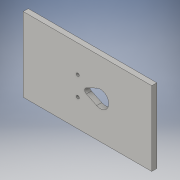
# Autodesk Inventor part: MOTORTOP
Saved by Autodesk Inventor 2016 (Build 200138000, 138)
## iProperties
Created: 2019-01-23
Part Number: MOTORTOP
Material: Generic
Document SubType Name: Modeling
Designer: student
Density: 1 g/cm^3
Appearance: Default
Author: student
Autodesk Inventor part; units mm, degrees
ref_plane "YZ Plane" through (0, 0, 0) normal (1, 0, 0) x (0, 1, 0)
ref_plane "XZ Plane" through (0, 0, 0) normal (0, 1, 0) x (-1, 0, 0)
ref_plane "XY Plane" through (0, 0, 0) normal (0, 0, 1) x (1, 0, 0)
sketch "Sketch1" plane through (0, 0, 0) normal (0, 0, 1) x (1, 0, 0)
  circle A0 centre (0, 0) radius 6.35 construction
  line L0 (0, 6.35) -> (-19.05, 6.35) construction
  circle A1 centre (-11.684, 0) radius 1.905 construction
  line L1 (-11.684, 0) -> (-19.05, 0) construction
  line L2 (-19.05, 0) -> (-20.3962, 0) construction
  line L3 (-20.3962, 0) -> (-20.3962, 7.4295) construction
  line L4 (-20.3962, 0) -> (-20.3962, -7.4295) construction
  line L5 (-20.3962, 7.4295) -> (-20.3962, 8.7757) construction
  circle A2 centre (-20.3962, 8.7757) radius 1.3462
  line L6 (-20.3962, -7.4295) -> (-20.3962, -8.7757) construction
  circle A3 centre (-20.3962, -8.7757) radius 1.3462
  arc A4 (-3.3157, -6.8608) -> (-4.2121, 6.35) centre (0, 0) ccw
  arc A5 (-12.6572, 2.3462) -> (-12.6572, -2.3462) centre (-11.684, 0) ccw
  line L7 (-12.6572, 2.3462) -> (-3.3157, 6.8608)
  line L8 (-12.6572, -2.3462) -> (-3.3157, -6.8608)
  line L9 (-69.6934, -33.5262) -> (46.3254, -33.5262)
  line L10 (46.3254, -33.5262) -> (46.3254, 33.5262)
  line L11 (46.3254, 33.5262) -> (-69.6934, 33.5262)
  line L12 (-69.6934, 33.5262) -> (-69.6934, -33.5262)
  dimension "d7" = 12.7
  dimension "d8" = 19.05
  dimension "d11" = 3.429
  dimension "d12" = 3.81
  dimension "d13" = 1.3462
  dimension "d14" = 7.4295
  dimension "d15" = 7.4295
  dimension "d16" = 1.3462
  dimension "d17" = 1.3462
  dimension "d18" = 15.24
  dimension "d19" = 5.08
  constraints: 26 end point, 5 horizontal, 5 point on circle, 4 coincident, 4 vertical, 3 centre point, 3 vertical alignment, 2 parallel, 2 tangent, 1 perpendicular, 1 point on line, 6 other
  measures "d8" distance of L0.start L0.end
  measures "d12" diameter of A1
  measures "d13" distance of L1.end L2.end
  measures "d14" distance of L2.end L3.end
  measures "d15" distance of L2.end L4.end
  measures "d16" distance of L3.end L5.end
  measures "d17" distance of L4.end L6.end
  measures "d18" diameter of A4
  measures "d19" diameter of A5
extrude "Extrusion1" add sketch "Sketch1" along normal blind 4.572
body "Solid1"
